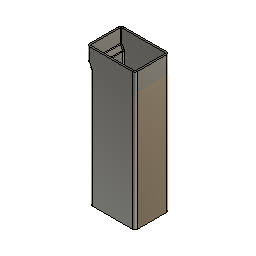
BatteryCase v1 (Autodesk Fusion 360 design; units mm, degrees)
Autodesk Fusion 360 part; units mm, degrees
sketch "Sketch1" plane through (0, 0, 0) normal (0, 0, 1) x (1, 0, 0)
  line L0 (22.5, 16.5) -> (-22.5, 16.5)
  line L1 (-22.5, 16.5) -> (-22.5, -16.5)
  line L2 (-22.5, -16.5) -> (22.5, -16.5)
  line L3 (22.5, -16.5) -> (22.5, 16.5)
  line L4 (22.5, 16.5) -> (-22.5, -16.5) construction
  line L5 (-22.5, 16.5) -> (22.5, -16.5) construction
  line L6 (24.4, 18.4) -> (-24.4, 18.4)
  line L7 (-24.4, 18.4) -> (-24.4, -18.4)
  line L8 (-24.4, -18.4) -> (24.4, -18.4)
  line L9 (24.4, -18.4) -> (24.4, 18.4)
  line L10 (24.4, 18.4) -> (-24.4, -18.4) construction
  line L11 (-24.4, 18.4) -> (24.4, -18.4) construction
  dimension "d1" = 45
  dimension "d2" = 33
  dimension "d3" = 1.9
  dimension "d4" = 1.9
  measures "d3" distance of L0 L6
  measures "d4" distance of L3 L9
extrude "Extrude1" add sketch "Sketch1" against normal blind 1.5 contours L0 L1 L2 L3 | L6 L7 L8 L9
extrude "Extrude2" add sketch "Sketch1" along normal blind 125
sketch "Sketch2" plane through (24.4, 0, 0) normal (1, 0, 0) x (0, 1, 0)
  line L0 (-18.4, 125) -> (-18.4, -1.5)
  line L1 (-18.4, -1.5) -> (18.4, -1.5)
  line L2 (18.4, -1.5) -> (18.4, 125)
  line L3 (18.4, 125) -> (-18.4, 125)
sketch "Sketch6" plane through (0, -18.4, 0) normal (0, -1, 0) x (1, 0, 0)
  line L0 (-24.4, 125) -> (-24.4, -1.5)
  line L1 (-24.4, -1.5) -> (24.4, -1.5)
  line L2 (24.4, -1.5) -> (24.4, 125)
  line L3 (24.4, 125) -> (-24.4, 125)
  line L4 (-24.4, 125) -> (-27.4, 130)
  line L5 (-27.4, 130) -> (-27.4, 145)
  line L6 (-27.4, 145) -> (-25.5, 145)
  line L7 (-25.5, 145) -> (-25.5, 130)
  line L8 (-25.5, 130) -> (-22.5, 125)
  line L9 (22.5, 0) -> (-22.5, 0)
  dimension "d26" = 130
  dimension "d27" = 145
  dimension "d28" = 3
  measures "d27" distance of L6 L9
extrude "Extrude6" add sketch "Sketch6" against normal up to surface (36.8 mm away) contours L3 L4 L5 L6 L7 L8
sketch "Sketch7" plane through (0, -18.4, 0) normal (0, -1, 0) x (1, 0, 0)
  line L0 (-24.4, 125) -> (-24.4, -1.5)
  line L1 (-24.4, -1.5) -> (24.4, -1.5)
  line L2 (24.4, -1.5) -> (24.4, 125)
  line L3 (24.4, 125) -> (-22.5, 125)
  line L4 (-22.5, 125) -> (-25.5, 130)
  line L5 (-25.5, 130) -> (-25.5, 145)
  line L6 (-25.5, 145) -> (-27.4, 145)
  line L7 (-27.4, 145) -> (-27.4, 130)
  line L8 (-27.4, 130) -> (-24.4, 125)
  line L9 (-25.5, 145) -> (24.4, 145)
  line L10 (24.4, 145) -> (24.4, 125)
extrude "Extrude7" add sketch "Sketch7" against normal up to surface (1.9 mm away) contours L3 L4 L5 L9 L10
ref_plane "WorkPlane1" through (-1.5, 0, 71.75) normal (0, -1, 0) x (-1, 0, 0)
mirror "Mirror1" about plane through (-1.5, 0, 71.75) normal (0, -1, 0) of "Extrude7"
extrude "Extrude8" add 1 faces at (23.7667, 5.5, 125) along direction (0, 0, 1) up to surface (20 mm away)
fillet "Fillet7" radius 1 2 edges at (-24.4, 0, 125) (-27.4, 0, 130)
fillet "Fillet8" radius 2 2 edges at (-22.5, 0, 125) (-25.5, 0, 130)
fillet "Fillet4" radius 2 4 edges at (0, 16.5, 0) (22.5, 0, 0) (0, -16.5, 0) (-22.5, 0, 0)
fillet "Fillet9" radius 1 16 edges at (-21.9142, 15.9142, 0.5858) (-22.5, 16.5, 63.223) (-22.5726, 16.5, 124.9799) (-24, 16.5, 127.5) (-25.4274, 16.5, 130.0201) (-25.5, 16.5, 137.777) (-25.5, -16.5, 137.777) (-25.4274, -16.5, 130.0201) (-24, -16.5, 127.5) (-22.5726, -16.5, 124.9799) (-22.5, -16.5, 63.223) (-21.9142, -15.9142, 0.5858) (21.9142, 15.9142, 0.5858) (22.5, 16.5, 73.5) (21.9142, -15.9142, 0.5858) (22.5, -16.5, 73.5)
fillet "Fillet10" radius 2.9 12 edges at (-24.4, 18.4, 61.6115) (-24.4363, 18.4, 124.9899) (-25.9, 18.4, 127.5) (-27.3637, 18.4, 130.0101) (-27.4, 18.4, 137.6385) (-24.4, -18.4, 61.6115) (-24.4363, -18.4, 124.9899) (-25.9, -18.4, 127.5) (-27.3637, -18.4, 130.0101) (-27.4, -18.4, 137.6385) (24.4, 18.4, 71.75) (24.4, -18.4, 71.75)
equation "d4 = d3"
